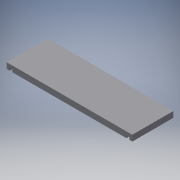
# Autodesk Inventor part: Door top
Saved by Autodesk Inventor 2016 (Build 200138000, 138)
## iProperties
Created: 2017-10-31
Part Number: Door top
Material: Wood (Oak)
Document SubType Name: Modeling
Designer: mathaetaes
Density: 0.76 g/cm^3
Appearance: White Oak - Natural Medium Gloss
Author: mathaetaes
Autodesk Inventor part; units mm, degrees
ref_plane "YZ Plane" through (0, 0, 0) normal (1, 0, 0) x (0, 1, 0)
ref_plane "XZ Plane" through (0, 0, 0) normal (0, 1, 0) x (-1, 0, 0)
ref_plane "XY Plane" through (0, 0, 0) normal (0, 0, 1) x (1, 0, 0)
sketch "Sketch1" plane through (0, 0, 0) normal (0, 1, 0) x (-1, 0, 0)
  line L0 (0, -133.35) -> (-407.9875, -133.35)
  line L1 (-407.9875, -133.35) -> (-407.9875, 0)
  line L2 (-407.9875, 0) -> (0, 0)
  line L3 (0, 0) -> (0, -133.35)
  dimension "d0" = 407.9875
  dimension "d1" = 133.35
  constraints: 8 end point, 2 parallel, 1 coincident, 1 horizontal, 1 perpendicular
  measures "d0" distance of L1.end L2.end
  measures "d1" distance of L0.end L1.end
extrude "Board" add sketch "Sketch1" along normal blind 19.05
sketch "Sketch2" plane through (0, 0, 0) normal (0, 0, 1) x (1, 0, 0)
  line L0 (19.05, 0) -> (9.525, 0)
  line L1 (9.525, 0) -> (9.525, 9.525)
  line L2 (9.525, 9.525) -> (19.05, 9.525)
  line L3 (19.05, 9.525) -> (19.05, 0)
  line L4 (0, 0) -> (0, 19.05) projected
  line L5 (407.9875, 0) -> (0, 0) projected
  line L6 (398.4625, 0) -> (388.9375, 0)
  line L7 (388.9375, 0) -> (388.9375, 9.525)
  line L8 (388.9375, 9.525) -> (398.4625, 9.525)
  line L9 (398.4625, 9.525) -> (398.4625, 0)
  line L10 (407.9875, 0) -> (407.9875, 19.05) projected
  dimension "d4" = 9.525
  dimension "d5" = 9.525
  dimension "d6" = 9.525
  dimension "d10" = 9.525
  constraints: 16 end point, 4 parallel, 2 collinear, 2 equal length, 2 horizontal, 2 perpendicular
  measures "d4" distance of L1.end L2.end
  measures "d5" distance of L0.end L1.end
  measures "d6" distance between parallel lines of L4 L1
  measures "d10" distance between parallel lines of L9 L10
extrude "Dado" cut sketch "Sketch2" against normal blind 133.35
equation "\"d0\" = DoorWidth"
equation "\"d10\" = d6"
equation "\"d7\" = d1"
equation "\"DoorWidth\" = 407.9875"
body "Solid1"
